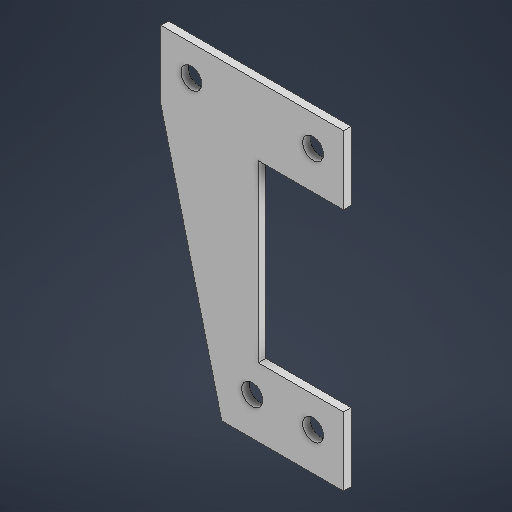
# Autodesk Inventor part: FrontFunnelBottom
Saved by Autodesk Inventor 2026.1 (Build 301233000, 233)
## iProperties
Created: 2025-08-03
Part Number: FrontFunnelBottom
Material: Generic
Document SubType Name: Modeling
Designer: roejo
Density: 1 g/cm^3
Appearance: Default
Author: roejo
Autodesk Inventor part; units mm, degrees
ref_plane "YZ Plane" through (0, 0, 0) normal (1, 0, 0) x (0, 1, 0)
ref_plane "XZ Plane" through (0, 0, 0) normal (0, 1, 0) x (-1, 0, 0)
ref_plane "XY Plane" through (0, 0, 0) normal (0, 0, 1) x (1, 0, 0)
sketch "Sketch1" plane through (0, 0, 0) normal (0, 0, 1) x (1, 0, 0)
  line L0 (-15.6363, 35.4419) -> (22.4637, 35.4419)
  line L1 (22.4637, 35.4419) -> (22.4637, 21.1544)
  line L2 (22.4637, -15.3581) -> (22.4637, -29.6456)
  line L3 (-2.9363, -29.6456) -> (-15.6363, 21.1544)
  line L4 (22.4637, 21.1544) -> (4.6837, 21.1544)
  line L5 (4.6837, 21.1544) -> (4.6837, -15.3581)
  line L6 (-15.6363, 35.4419) -> (-15.6363, 21.1544)
  line L7 (22.4637, -15.3581) -> (4.6837, -15.3581)
  line L8 (22.4637, -29.6456) -> (-2.9363, -29.6456)
  circle A0 centre (16.1137, 29.0919) radius 2.1844
  circle A1 centre (-9.2863, 29.0919) radius 2.1844
  circle A2 centre (16.1137, -21.7081) radius 2.1844
  circle A3 centre (3.4137, -21.7081) radius 2.1844
  point P0 (0, 0)
  dimension "d0" = 38.1
  dimension "d1" = 17.78
  constraints: 18 end point, 4 centre point, 2 point on line, 1 horizontal, 1 parallel, 1 vertical
  measures "d0" distance of L0.start L0.end
  measures "d1" distance of L1.end L4.end
extrude "Extrusion1" add sketch "Sketch1" along normal blind 1.5875
body "Solid1"
